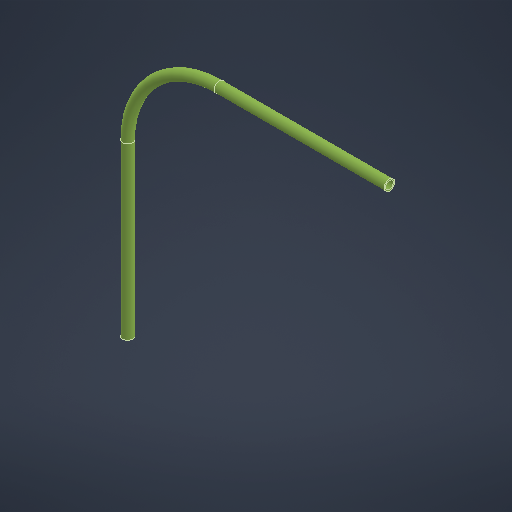
# Autodesk Inventor part: TorsionOscillator-FillLine-Coupling
Saved by Autodesk Inventor 2026 (Build 300175050, 175E)
## iProperties
Created: 2023-08-18
Part Number: TorsionOscillator-FillLine-Coupling
Material: Nickel-Copper Alloy 400
Document SubType Name: Modeling
Designer: schanen
Density: 8.83 g/cm^3
Appearance: Olive Green
Author: schanen
Autodesk Inventor part; units mm, degrees
ref_plane "YZ Plane" through (0, 0, 0) normal (1, 0, 0) x (0, 1, 0)
ref_plane "XZ Plane" through (0, 0, 0) normal (0, 1, 0) x (-1, 0, 0)
ref_plane "XY Plane" through (0, 0, 0) normal (0, 0, 1) x (1, 0, 0)
sketch "Sketch1" plane through (0, 0, 0) normal (0, 0, 1) x (1, 0, 0)
  line L0 (7, 20) -> (20, 20)
  line L1 (0, 13) -> (0, 0)
  arc A0 (7, 20) -> (0, 13) centre (7, 13) ccw
  dimension "d3" = 7
  dimension "d10" = 20
  dimension "d11" = 20
  constraints: 4 end point, 2 point on circle, 1 centre point, 1 coincident, 1 horizontal, 1 horizontal alignment, 1 vertical, 1 vertical alignment
  measures "d3" radius of A0
  measures "d10" distance from line of L0.end L1
  measures "d11" distance from line of L1.end L0
sketch "Sketch2" plane through (0, 0, 0) normal (0, 1, 0) x (-1, 0, 0)
  circle A0 centre (0, 0) radius 0.4
  circle A1 centre (0, 0) radius 0.3
  dimension "d6" = 0.8
  dimension "d9" = 0.6
  constraints: 2 centre point, 2 coincident
  measures "d6" diameter of A0
  measures "d9" diameter of A1
sweep "Sweep1" add profiles "Sketch2" path "Sketch1"
body "Solid1"
